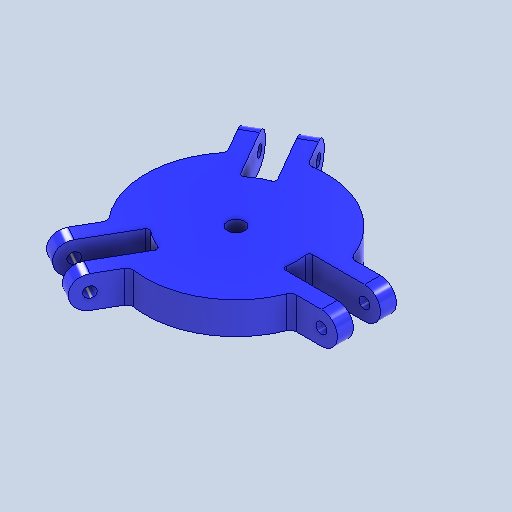
# Autodesk Inventor part: hand-grab-v1-3DP-link-F-2
Saved by Autodesk Inventor 2025.2 (Build 292293000, 293)
## iProperties
Created: 2024-10-07
Part Number: hand-grab-v1-3DP-link-F-2
Material: ABS プラスチック
Document SubType Name: Modeling
Designer: haruy
Density: 1.06 g/cm^3
Appearance: 青 - 壁塗料 - 光沢
Author: haruy
Autodesk Inventor part; units mm, degrees
ref_plane "YZ Plane" through (0, 0, 0) normal (1, 0, 0) x (0, 1, 0)
ref_plane "XZ Plane" through (0, 0, 0) normal (0, 1, 0) x (-1, 0, 0)
ref_plane "XY Plane" through (0, 0, 0) normal (0, 0, 1) x (1, 0, 0)
derived "hand-grab-v1-Sketch-Base.ipt"
sketch "スケッチ1" plane through (400, 0, 0) normal (1, 0, 0) x (0, 1, 0)
  circle A0 centre (0, 0) radius 120
  circle A1 centre (-109.552214, 63.25) radius 6.5
  line L0 (0, 0) -> (-109.552214, 63.25)
  line L1 (0, 0) -> (0, 120)
  line L2 (246.086224, 200) -> (-251.460254, 200)
  circle A2 centre (145, 60) radius 254.57296
  circle A3 centre (-67.6203, 200) radius 6.5
  line L3 (0, 0) -> (-120, 0)
  line L4 (249, 9.15) -> (187, 9.15)
  line L5 (187, 9.15) -> (187, -9.15)
  line L6 (187, -9.15) -> (249, -9.15)
  line L7 (249, -9.15) -> (249, 9.15)
  line L8 (187, 5.15) -> (179, 5.15)
  line L9 (179, 5.15) -> (179, -4.85)
  line L10 (179, -4.85) -> (187, -4.85)
  line L11 (187, -4.85) -> (187, 5.15)
  line L12 (179, 3.15) -> (174, 3.15)
  line L13 (174, 3.15) -> (174, -2.85)
  line L14 (174, -2.85) -> (179, -2.85)
  line L15 (179, -2.85) -> (179, 3.15)
  line L16 (174, 2.65) -> (159, 2.65)
  line L17 (159, 2.65) -> (159, -2.35)
  line L18 (159, -2.35) -> (174, -2.35)
  line L19 (174, -2.35) -> (174, 2.65)
  line L20 (187, 34.15) -> (184, 34.15)
  line L21 (184, 34.15) -> (184, -43.518169)
  line L22 (184, -43.518169) -> (187, -43.518169)
  line L23 (187, -43.518169) -> (187, 34.15)
  circle A4 centre (150, 65) radius 4
  circle A5 centre (150, 65) radius 14
  line L24 (187, 34.15) -> (192, 34.15)
  line L25 (192, 34.15) -> (192, 14.15)
  line L26 (192, 14.15) -> (187, 14.15)
  line L27 (187, 14.15) -> (187, 34.15)
  line L28 (184, 34.15) -> (147.580449, 61.814757)
  line L29 (151.353345, 68.764101) -> (192, 54.15)
  line L30 (192, 54.15) -> (192, 34.15)
  line L31 (239.386769, 130) -> (-239.386769, 130)
  circle A6 centre (-109.552214, 63.25) radius 4
  circle A7 centre (150, 65) radius 9
  line L32 (-106.088112, 61.25) -> (-113.016315, 65.25)
  line L33 (170, 36) -> (155, 36)
  circle A8 centre (155, 36) radius 5
  circle A9 centre (155, 36) radius 9
  circle A10 centre (-90.698003, 156.1969) radius 6.5
  circle A11 centre (170, 36) radius 5
  line L34 (150, 65) -> (170, 36)
  circle A12 centre (170, 36) radius 9
  circle A13 centre (150, 65) radius 44.22783
  line L35 (150, 65) -> (155, 36)
  line L36 (150, 65) -> (-109.552214, 63.25)
  line L37 (-90.698003, 156.1969) -> (150, 65)
  line L38 (150, 65) -> (157.514614, 21.415238)
  circle A14 centre (150, 65) radius 35.22783
  circle A15 centre (155.985452, 30.284379) radius 9
  line L39 (168.077664, 21.284379) -> (136, 21.284379)
  line L40 (175, 3.15) -> (175, -2.85)
  point P0 (-60, 0)
sketch "スケッチ2" plane through (0, 400, 0) normal (0, 1, 0) x (-1, 0, 0)
  circle A0 centre (0, 0) radius 120
  line L0 (0, 0) -> (-331.462521, 0)
  line L1 (67.5, -116.91343) -> (-135, 0)
  circle A1 centre (0, 0) radius 5.1
  line L2 (0, 0) -> (67.5, 116.91343)
  line L3 (0, 0) -> (67.5, -116.91343)
  line L4 (0, 0) -> (-135, 0)
  line L5 (17.035898, 37.507042) -> (12.035898, 28.846788)
  line L6 (12.035898, 28.846788) -> (15.5, 26.846788)
  line L7 (15.5, 26.846788) -> (20.5, 35.507042)
  line L8 (20.5, 35.507042) -> (17.035898, 37.507042)
  line L9 (20.5, 35.507042) -> (15.5, 26.846788)
  line L10 (15.5, 26.846788) -> (18.964102, 24.846788)
  line L11 (18.964102, 24.846788) -> (23.964102, 33.507042)
  line L12 (23.964102, 33.507042) -> (20.5, 35.507042)
  line L13 (14.535898, 33.176915) -> (21.464102, 29.176915)
  circle A2 centre (0, 0) radius 2.65
  line L14 (16.819392, 37.632042) -> (10.319392, 26.373711)
  line L15 (10.319392, 26.373711) -> (5.989265, 28.873711)
  line L16 (5.989265, 28.873711) -> (12.489265, 40.132042)
  line L17 (12.489265, 40.132042) -> (16.819392, 37.632042)
  line L18 (28.510735, 30.882042) -> (24.180608, 33.382042)
  line L19 (22.010735, 19.623711) -> (28.510735, 30.882042)
  line L20 (24.180608, 33.382042) -> (17.680608, 22.123711)
  line L21 (17.680608, 22.123711) -> (22.010735, 19.623711)
  circle A3 centre (0, 0) radius 28.320708
  line L22 (-41, 9.25) -> (-41, 4.25)
  line L23 (-41, 4.25) -> (-28, 4.25)
  line L24 (-28, 9.25) -> (-41, 9.25)
  line L25 (-28, 4.25) -> (-28, 9.25)
  line L26 (-41, -4.25) -> (-28, -4.25)
  line L27 (-41, -9.25) -> (-41, -4.25)
  line L28 (-28, -9.25) -> (-41, -9.25)
  line L29 (-28, -4.25) -> (-28, -9.25)
  line L30 (12.489265, -40.132042) -> (16.819392, -37.632042)
  line L31 (16.819392, -37.632042) -> (10.319392, -26.373711)
  line L32 (5.989265, -28.873711) -> (12.489265, -40.132042)
  line L33 (10.319392, -26.373711) -> (5.989265, -28.873711)
  line L34 (24.180608, -33.382042) -> (17.680608, -22.123711)
  line L35 (28.510735, -30.882042) -> (24.180608, -33.382042)
  line L36 (22.010735, -19.623711) -> (28.510735, -30.882042)
  line L37 (17.680608, -22.123711) -> (22.010735, -19.623711)
  line L38 (5.989265, 28.873711) -> (5.373024, 27.80635)
  line L39 (22.010735, 19.623711) -> (21.394494, 18.55635)
  line L40 (-28, 9.25) -> (-26.767518, 9.25)
  line L41 (-28, -9.25) -> (-26.767518, -9.25)
  line L42 (5.989265, -28.873711) -> (2.193431, -22.299134)
  line L43 (22.010735, -19.623711) -> (21.394494, -18.55635)
  line L44 (13.610898, 31.574768) -> (3.610898, 14.254259) construction
  line L45 (3.610898, 14.254259) -> (-1.585254, 17.254259) construction
  line L46 (-1.585254, 17.254259) -> (8.414746, 34.574768) construction
  line L47 (8.414746, 34.574768) -> (13.610898, 31.574768) construction
  circle A4 centre (3.512822, 20.084386) radius 1.6 construction
  circle A5 centre (8.512822, 28.744641) radius 1.6 construction
  circle A6 centre (20.637178, 21.744641) radius 1.6 construction
  circle A7 centre (15.637178, 13.084386) radius 1.6 construction
  circle A8 centre (-29.15, 7) radius 1.6 construction
  circle A9 centre (-19.15, 7) radius 1.6 construction
  circle A10 centre (-19.15, -7) radius 1.6 construction
  circle A11 centre (-29.15, -7) radius 1.6 construction
  circle A12 centre (8.512822, -28.744641) radius 1.6 construction
  circle A13 centre (3.512822, -20.084386) radius 1.6 construction
  circle A14 centre (15.637178, -13.084386) radius 1.6 construction
  circle A15 centre (20.637178, -21.744641) radius 1.6 construction
  line L48 (1.012822, 15.754259) -> (13.610898, 31.574768) construction
  circle A16 centre (0, 0) radius 34.383463
  circle A17 centre (0, 0) radius 19
  line L49 (21.394494, 18.55635) -> (16.30889, 9.747826)
  line L50 (17.680608, 22.123711) -> (12.939894, 13.912554)
  line L51 (10.319392, 26.373711) -> (5.578678, 18.162554)
  line L52 (5.373024, 27.80635) -> (0.28742, 18.997826)
  line L53 (-8, 47) -> (-188, 47)
  line L54 (-188, 47) -> (-188, 32)
  line L55 (-188, 32) -> (-8, 32)
  line L56 (-8, 32) -> (-8, 47)
  point P0 (-28, -4.25)
  point P1 (5.373024, -27.80635)
  point P2 (10.319392, -26.373711)
  point P3 (17.680608, -22.123711)
  point P4 (17.680608, 22.123711)
  point P5 (17.680608, 22.123711)
  dimension "d19" = 38
  measures "d19" diameter of A17
ref_plane "作業平面1" through (400, 0, 0) normal (1, 0, 0) x (0, 1, 0)
ref_plane "作業平面2" through (0, 400, 0) normal (0, 1, 0) x (-1, 0, 0)
extrude "押し出し1" add sketch "スケッチ2" along normal blind 10 contours A3 L0 A17 L3 | L3 A17 L49 A3 | A16 L32 L33 L31 | L31 L30 L32 A16 | A16 L36 L35 L34 | L34 L37 L36 A16 | A17 L0 A1 L3 | L3 A1 L2 A17 | L33 L42 A3 | A3 L43 L37 | A16 L23 L22 L24 | L24 L25 L23 A16 | A16 L14 L15 L16 | L16 L17 L14 A16 | L3 A2 L2 A1 | A1 L0 A2 L3 | A17 L2 A1 L0 | L0 A3 L52 A17 | A16 L26 L29 L28 | L28 L27 L26 A16 | L40 A3 L25 | L15 A3 L38 | A3 L50 A17 L2 | L2 A17 L51 A3 | A16 L19 L21 L20 | L20 L18 L19 A16 | A1 L2 A2 L0 | L52 A3 L51 A17 | A17 L50 A3 L49 | L41 L29 A3 | L21 L39 A3
sketch "スケッチ3" plane through (-5.373024, 400, 27.80635) normal (0.8660254, 0, 0.5) x (0.5, 0, -0.8660254)
  line L0 (-14.232482, 0) -> (-14.232482, 10)
  line L1 (-390.953758, 0) -> (526.310378, 0)
  point P0 (26.767518, -400)
  point P1 (-9.232482, 5)
  dimension "d3" = 5
  dimension "d4" = 5
  measures "d3" distance from line of point (-9.232, 5) L0
  measures "d4" distance from line of L1 point (-9.232, 5)
hole "穴1" at (-9.989265, 405, 35.801915) direction (-0.8660254, 0, -0.5) diameter 3.4 end through all
pattern_circular "円形状パターン1" count 3 over 360 about axis through (0, 400, 0) along (0, 1, 0) of "穴1"
extrude "押し出し2" cut sketch "スケッチ2" along normal blind 10 contours A3 L50 A17 L2 | L2 A17 L51 A3
pattern_circular "円形状パターン3" count 3 over 360 about axis through (0, 400, 0) along (0, 1, 0) of "押し出し2"
fillet "フィレット2" radius 1 2 edges at (-5.5787, 405, 18.1626) (-12.9399, 405, 13.9126)
fillet "フィレット3" radius 2 2 edges at (-21.3945, 405, 18.5564) (-5.373, 405, 27.8064)
pattern_circular "円形状パターン4" count 3 over 360 about axis through (0, 400, 0) along (0, 1, 0) of "フィレット2", "フィレット3"
sketch "スケッチ4" plane through (-22.088935, 400, 19.759157) normal (-0.8660254, 0, -0.5) x (-0.5, 0, 0.8660254)
  circle A0 centre (7.843601, 5) radius 1.7
  circle A1 centre (7.843601, 5) radius 5
  line L0 (12.843601, 0) -> (12.843601, 10)
  line L1 (12.843601, 10) -> (0, 10)
  line L2 (12.843601, 0) -> (3.493831, 0)
  line L3 (3.493831, 0) -> (3.493831, 10)
  line L4 (3.493831, 10) -> (12.843601, 10)
  line L5 (12.843601, 10) -> (12.843601, 0)
  point P0 (-28.156399, -400)
  point P1 (10.843601, 10)
  point P2 (12.843601, 10)
  point P3 (7.843601, 10)
  point P4 (12.843601, 5)
  point P5 (7.843601, 0)
  dimension "d30" = 10
  constraints: 8 end point, 2 parallel, 1 centre point, 1 coincident, 1 horizontal, 1 perpendicular, 1 point on line
  measures "d30" diameter of A1
extrude "押し出し3" cut sketch "スケッチ4" against normal through all contours L0 L2 A1 | A1 L1 L0
pattern_circular "円形状パターン5" count 3 over 360 about axis through (0, 400, 0) along (0, 1, 0) of "押し出し3"
